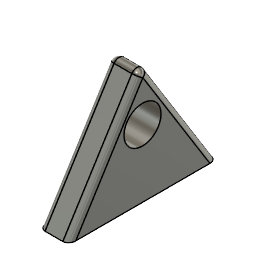
Base Hydra 1.3 (Autodesk Fusion 360 archive; units mm, degrees)
design "Pivot Joint"
part number: 2026-07-24-22-20-55-985
Autodesk Fusion 360 part; units mm, degrees
sketch "Sketch1" plane through (0, 0, 0) normal (1, 0, 0) x (0, 0, -1)
  line L0 (-20, 0) -> (30, 0)
  line L1 (30, 0) -> (5, 40.1542)
  line L2 (5, 40.1542) -> (-20, 0)
  constraint horizontal L0
extrude "Extrude1" add sketch "Sketch1" along normal blind 10
fillet "Fillet1" radius 2 5 edges at (5, 40.1542, -5) (10, 20.0771, 7.5) (10, 20.0771, -17.5) (0, 20.0771, -17.5) (0, 20.0771, 7.5)
hole "Hole1" at (10, 22.7245, -4.8931) direction (-1, 0, 0) diameter 12.5 depth 700 tip angle 118

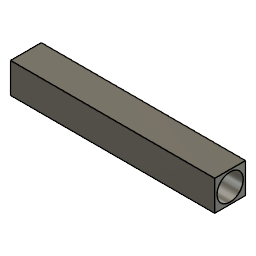
design "shoulder"
part number: 2026-07-24-22-13-45-032
Autodesk Fusion 360 part; units mm, degrees
sketch "Sketch1" plane through (0, 0, 0) normal (0, 1, 0) x (1, 0, 0)
  line L0 (-200, -50) -> (150, -50)
  line L1 (150, -50) -> (150, 2.8514)
  line L2 (150, 2.8514) -> (-200, 2.8514)
  line L3 (-200, 2.8514) -> (-200, -50)
  dimension "d1" = 350
  constraint horizontal L0
  constraint vertical L1
  constraint horizontal L2
  constraint vertical L3
  measures "d1" distance of L0.start L0.end
extrude "Extrude1" add sketch "Sketch1" along normal blind 52
hole "Hole1" at (-200, 26, 23.5743) direction (1, 0, 0) diameter 45 depth 700 tip angle 118

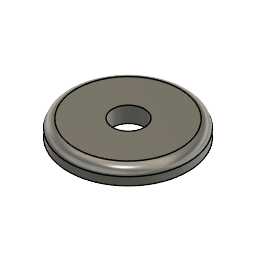
design "Untitled"
part number: 2026-07-24-15-04-10-705
Autodesk Fusion 360 part; units mm, degrees
cylinder "CylinderPrimitive1" add diameter 150 height 20 placed x (1, 0, 0) y (0, 0, -1) z (0, 1, 0) at (0, 0, 0)
fillet "Fillet1" radius 10 1 edges at (-69.9246, 20, 27.1212)
sketch "Sketch2" plane through (0, 0, 0) normal (1, 0, 0) x (0, 0, -1)
hole "Hole1" at (-0.3862, 20, -1.0042) direction (0, -1, 0) diameter 40 depth 60 tip angle 180
sketch "Sketch3" plane through (0, 0, 0) normal (0, 0, 1) x (1, 0, 0)

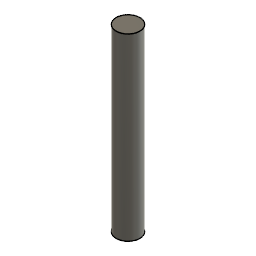
design "hydra stopper"
part number: 2026-07-27-21-17-18-488
Autodesk Fusion 360 part; units mm, degrees
cylinder "CylinderPrimitive1" add diameter 12.5 height 94.32 placed x (1, 0, 0) y (0, 0, -1) z (0, 1, 0) at (-4.815, 0, 0)

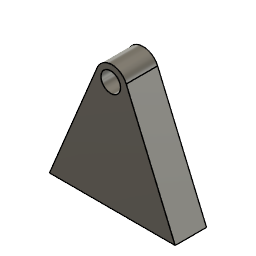
design "Clewis Bracket 1.2"
part number: 2026-07-24-20-30-49-750
Autodesk Fusion 360 part; units mm, degrees
sketch "Sketch1" plane through (0, 0, 0) normal (0, 0, 1) x (1, 0, 0)
  line L0 (-40, 0) -> (-0.4355, 95.3806)
  line L1 (-0.4355, 95.3806) -> (40, 0)
  line L2 (40, 0) -> (-40, 0)
  constraint horizontal L2
extrude "Extrude1" add sketch "Sketch1" along normal blind 20
hole "Hole1" at (-0.9754, 69.5316, 20) direction (0, 0, -1) diameter 12.5 depth 40 tip angle 118
fillet "Fillet1" radius 10 1 edges at (-0.4355, 95.3806, 10)
